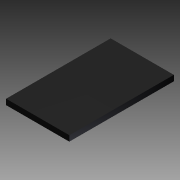
# Autodesk Inventor part: Nexus7
Saved by Autodesk Inventor 2012 (Build 160160000, 160)
## iProperties
Created: 2013-07-14
Part Number: Nexus7
Material: Default
Document SubType Name: Modeling
Designer: joe_000
Density: 1.35168 g/cm^3
Mass: 340 g
Surface Area: 543.667 cm^2
Volume: 251.539 cm^3
TabletHeight: 198.500 mm
TabletWidth: 120.000 mm
TabletThickness: 10.560 mm
Author: joe_000
Autodesk Inventor part; units mm, degrees
ref_plane "YZ Plane" through (0, 0, 0) normal (1, 0, 0) x (0, 1, 0)
ref_plane "XZ Plane" through (0, 0, 0) normal (0, 1, 0) x (-1, 0, 0)
ref_plane "XY Plane" through (0, 0, 0) normal (0, 0, 1) x (1, 0, 0)
sketch "Sketch1" plane through (0, 0, 0) normal (0, 0, 1) x (1, 0, 0)
  line L0 (0, 0) -> (120, 0)
  line L1 (120, 0) -> (120, 198.5)
  line L2 (120, 198.5) -> (0, 198.5)
  line L3 (0, 198.5) -> (0, 0)
  dimension "TabletHeight" = 198.5
  dimension "TabletWidth" = 120
  constraints: 8 end point, 2 parallel, 1 horizontal, 1 perpendicular
  measures "TabletHeight" distance of L0.end L1.end
  measures "TabletWidth" distance of L1.end L2.end
extrude "Extrusion1" add sketch "Sketch1" along normal blind 10.56
body "Solid1"
